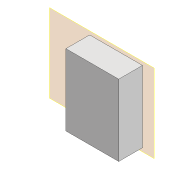
# Autodesk Inventor part: Base_isolante
Saved by Autodesk Inventor 2020 (Build 240168000, 168)
## iProperties
Created: 2022-07-16
Part Number: Base_isolante
Material: Genérico
Document SubType Name: Modeling
Designer: gabri
Density: 1 g/cm^3
Appearance: Padrão
Author: gabri
Autodesk Inventor part; units mm, degrees
ref_plane "YZ Plane" through (0, 0, 0) normal (1, 0, 0) x (0, 1, 0)
ref_plane "XZ Plane" through (0, 0, 0) normal (0, 1, 0) x (-1, 0, 0)
ref_plane "XY Plane" through (0, 0, 0) normal (0, 0, 1) x (1, 0, 0)
ref_plane "Plano de trabalho1" through (0, 0, 0) normal (0, 0, 1) x (1, 0, 0)
sketch "Esboço1" plane through (0, 0, 0) normal (0, 0, 1) x (1, 0, 0)
  arc A0 (98, -75) -> (100, -73) centre (98, -73) ccw projected
  line L0 (100, -73) -> (100, 73) projected
  arc A1 (100, 73) -> (98, 75) centre (98, 73) ccw projected
  line L1 (98, 75) -> (-98, 75) projected
  arc A2 (-98, 75) -> (-100, 73) centre (-98, 73) ccw projected
  line L2 (-100, 73) -> (-100, -73) projected
  arc A3 (-100, -73) -> (-98, -75) centre (-98, -73) ccw projected
  line L3 (-98, -75) -> (98, -75) projected
  line L4 (-25.7219, -75) -> (85.393, -75)
  line L5 (85.393, -75) -> (85.393, 75)
  line L6 (85.393, 75) -> (-25.7219, 75)
  line L7 (-25.7219, 75) -> (-25.7219, -75)
  point P0 (0, 0)
  constraints: 8 end point, 2 parallel, 2 point on line, 1 horizontal, 1 perpendicular
extrude "Extrusão1" add sketch "Esboço1" along normal blind 50 contours L3 L7 L1 L5
